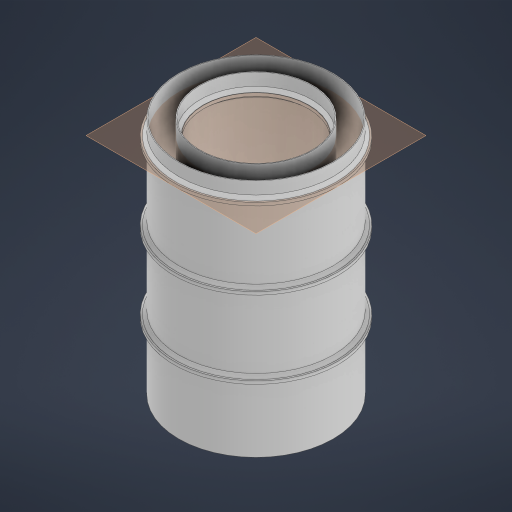
# Autodesk Inventor part: PechFormaTube
Saved by Autodesk Inventor 2024 (Build 280153000, 153)
## iProperties
Created: 2023-12-11
Part Number: PechFormaTube
Material: Generic
Document SubType Name: Modeling
Designer: KirikDK
Mass: 458.449 g
Surface Area: 6942.45 cm^2
Volume: 458.449 cm^3
Density: 1 g/cm^3
Appearance: Default
Author: KirikDK
Autodesk Inventor part; units mm, degrees
ref_plane "YZ Plane" through (0, 0, 0) normal (1, 0, 0) x (0, 1, 0)
ref_plane "XZ Plane" through (0, 0, 0) normal (0, 1, 0) x (-1, 0, 0)
ref_plane "XY Plane" through (0, 0, 0) normal (0, 0, 1) x (1, 0, 0)
sketch "Sketch1" plane through (0, 0, 0) normal (0, 1, 0) x (-1, 0, 0)
  circle A0 centre (0, 0) radius 72.5
  circle A1 centre (0, 0) radius 100
  circle A2 centre (0, -86) radius 2
  circle A3 centre (14.9337, -84.6935) radius 2
  circle A4 centre (29.4137, -80.8136) radius 2
  circle A5 centre (43, -74.4782) radius 2
  circle A6 centre (55.2797, -65.8798) radius 2
  circle A7 centre (65.8798, -55.2797) radius 2
  circle A8 centre (74.4782, -43) radius 2
  circle A9 centre (80.8136, -29.4137) radius 2
  circle A10 centre (84.6935, -14.9337) radius 2
  circle A11 centre (86, 0) radius 2
  circle A12 centre (84.6935, 14.9337) radius 2
  circle A13 centre (80.8136, 29.4137) radius 2
  circle A14 centre (74.4782, 43) radius 2
  circle A15 centre (65.8798, 55.2797) radius 2
  circle A16 centre (55.2797, 65.8798) radius 2
  circle A17 centre (43, 74.4782) radius 2
  circle A18 centre (29.4137, 80.8136) radius 2
  circle A19 centre (14.9337, 84.6935) radius 2
  circle A20 centre (0, 86) radius 2
  circle A21 centre (-14.9337, 84.6935) radius 2
  circle A22 centre (-29.4137, 80.8136) radius 2
  circle A23 centre (-43, 74.4782) radius 2
  circle A24 centre (-55.2797, 65.8798) radius 2
  circle A25 centre (-65.8798, 55.2797) radius 2
  circle A26 centre (-74.4782, 43) radius 2
  circle A27 centre (-80.8136, 29.4137) radius 2
  circle A28 centre (-84.6935, 14.9337) radius 2
  circle A29 centre (-86, 0) radius 2
  circle A30 centre (-84.6935, -14.9337) radius 2
  circle A31 centre (-80.8136, -29.4137) radius 2
  circle A32 centre (-74.4782, -43) radius 2
  circle A33 centre (-65.8798, -55.2797) radius 2
  circle A34 centre (-55.2797, -65.8798) radius 2
  circle A35 centre (-43, -74.4782) radius 2
  circle A36 centre (-29.4137, -80.8136) radius 2
  circle A37 centre (-14.9337, -84.6935) radius 2
  dimension "d0" = 145
  dimension "d1" = 200
  dimension "d7" = 360
  constraints: 38 centre point, 2 coincident, 73 other
  measures "d0" diameter of A0
  measures "d1" diameter of A1
extrude "Extrusion1" add sketch "Sketch1" along normal blind 310
shell "Shell1" thickness 1 removed faces 1 at (-11.5508, 310, -94.9198)
sketch "Sketch2" plane through (0, 0, 0) normal (0, -1, 0) x (1, 0, 0)
  circle A0 centre (0, 0) radius 72.5
  circle A1 centre (0, 0) radius 71.8694
  circle A2 centre (0, 0) radius 74.247
  circle A3 centre (0, 0) radius 98.333
  circle A4 centre (0, 0) radius 100.5055
  constraints: 5 centre point, 5 coincident
sketch "Sketch4" plane through (0, 310, 0) normal (0, 1, 0) x (1, 0, 0)
  circle A0 centre (0, 0) radius 73.5
  circle A1 centre (0, 0) radius 99
  dimension "d11" = 147
  dimension "d12" = 198
  constraints: 2 centre point, 2 coincident
  measures "d11" diameter of A0
  measures "d12" diameter of A1
extrude "Extrusion2" cut sketch "Sketch4" against normal blind 320
sketch "Sketch5" plane through (0, 310, 0) normal (0, 1, 0) x (1, 0, 0)
  circle A0 centre (0, 0) radius 72.1313
  circle A1 centre (0, 0) radius 71
  circle A2 centre (0, 0) radius 102
  circle A3 centre (0, 0) radius 100.2533
  constraints: 4 centre point, 4 coincident
extrude "Extrusion3" [suppressed]
sketch "Sketch6" plane through (0, 310, 0) normal (0, 1, 0) x (1, 0, 0)
  circle A0 centre (0, 0) radius 73
  circle A1 centre (0, 0) radius 71.4438
  circle A2 centre (0, 0) radius 99.5789
  circle A3 centre (0, 0) radius 101
  constraints: 4 centre point, 4 coincident
extrude "Extrusion4" [suppressed]
chamfer "Chamfer1" [suppressed]
chamfer "Chamfer2" [suppressed]
ref_plane "Work Plane1" through (0, 290, 0) normal (0, 1, 0) x (1, 0, 0)
sketch "Sketch7" plane through (0, 290, 0) normal (0, 1, 0) x (1, 0, 0)
  circle A0 centre (0, 0) radius 72.5
  circle A1 centre (0, 0) radius 68
  circle A2 centre (0, 0) radius 106
  circle A3 centre (0, 0) radius 100
  constraints: 4 centre point, 4 coincident
extrude "Extrusion5" add sketch "Sketch7" against normal blind 4
chamfer "Chamfer3" distance 4 angle 45 4 edges at (72.5, 290, 0) (100, 290, 0) (100, 286, 0) (72.5, 286, 0)
pattern_linear "Rectangular Pattern1" count 3 spacing 100 along (0, -1, 0) of "Extrusion5", "Chamfer3"
body "Solid1"
